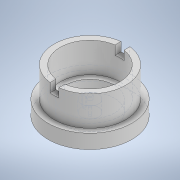
# Autodesk Inventor part: LidBottom
Saved by Autodesk Inventor 2020 (Build 240168000, 168)
## iProperties
Created: 2022-03-01
Part Number: LidBottom
Material: Generic
Document SubType Name: Modeling
Designer: atharun
Density: 1 g/cm^3
Appearance: Default
Mass: 115.288 g
Surface Area: 338.563 cm^2
Volume: 115.288 cm^3
Author: atharun
Autodesk Inventor part; units mm, degrees
sketch "Sketch1" plane through (0, 0, 0) normal (0, 1, 0) x (-1, 0, 0)
  circle A0 centre (0, 0) radius 44.45
  circle A1 centre (0, 0) radius 6.75
  dimension "d0" = 88.9
  dimension "d3" = 13.5
  constraints: 2 centre point, 2 coincident
  measures "d0" diameter of A0
  measures "d3" diameter of A1
extrude "Extrusion2" add sketch "Sketch1" along normal blind 2 contours A0 | A1
sketch "Sketch2" plane through (0, 2, 0) normal (0, 1, 0) x (1, 0, 0)
  circle A0 centre (0, 0) radius 10
  circle A1 centre (0, 0) radius 44.45
  dimension "d6" = 20
  dimension "d37" = 88.9
  constraints: 2 centre point, 2 coincident
  measures "d6" diameter of A0
  measures "d37" diameter of A1
extrude "Extrusion3" add sketch "Sketch2" along normal blind 7 contours A0 | A1
sketch "Sketch3" plane through (0, 9, 0) normal (0, 1, 0) x (1, 0, 0)
  circle A0 centre (0, 0) radius 44.45
  dimension "d9" = 88.9
  constraints: 1 centre point, 1 coincident
  measures "d9" diameter of A0
extrude "Extrusion4" add sketch "Sketch3" along normal blind 6
sketch "Sketch4" plane through (0, 15, 0) normal (0, 1, 0) x (1, 0, 0)
  circle A0 centre (0, 0) radius 38.0048
  circle A1 centre (0, 0) radius 31.75
  point P0 (-38.0048, 0)
  point P1 (0, 38.0048)
  point P2 (38.0048, 0)
  point P3 (0, -38.0048)
  dimension "d12" = 76.0095
  dimension "d13" = 63.5
  constraints: 4 point on circle, 2 centre point, 2 coincident
  measures "d12" diameter of A0
  measures "d13" diameter of A1
extrude "Extrusion5" add sketch "Sketch4" along normal blind 31.75
ref_plane "Work Plane3" through (38.0048, 15, 0) normal (1, 0, 0) x (0, 1, 0)
ref_plane "Work Plane4" through (-38.0048, 15, 0) normal (-1, 0, 0) x (0, -1, 0)
sketch "Sketch8" plane through (38.0048, 15, 0) normal (1, 0, 0) x (0, 1, 0)
  line L0 (31.75, -38.0048) -> (31.75, 38.0048) projected
  line L1 (31.75, 6.35) -> (14.224, 6.35)
  line L2 (14.224, 6.35) -> (14.224, -6.35)
  line L3 (14.224, -6.35) -> (31.75, -6.35)
  line L4 (31.75, -6.35) -> (31.75, 6.35)
  line L5 (31.75, 0) -> (0, 0)
  line L6 (0, -44.45) -> (0, 44.45) projected
  line L7 (21.844, 5.08) -> (17.4498, 5.08)
  line L8 (17.4498, 5.08) -> (17.4498, -5.08)
  line L9 (17.4498, -5.08) -> (21.844, -5.08)
  line L10 (21.844, -5.08) -> (21.844, 5.08)
  line L11 (25.146, 6.35) -> (25.146, -6.35)
  point P0 (-15, 0)
  dimension "d38" = 17.526
  dimension "d39" = 12.7
  dimension "d41" = 6.35
  dimension "d42" = 9.906
  dimension "d43" = 10.16
  dimension "d44" = 5.08
  dimension "d46" = 4.3942
  dimension "d70" = 6.604
  constraints: 20 end point, 4 parallel, 3 perpendicular, 3 point on line, 2 horizontal, 2 midpoint
  measures "d38" distance of L3.end L2.end
  measures "d39" distance of L2.end L1.end
  measures "d41" distance between parallel lines of L1 L5
  measures "d42" distance between parallel lines of L10 L0
  measures "d43" distance of L7.end L8.end
  measures "d44" distance between parallel lines of L5 L9
  measures "d46" distance of L7.start L7.end
  measures "d70" distance between parallel lines of L0 L11
extrude "Extrusion9" [suppressed]
ref_plane "Work Plane5" through (0, 15, 0) normal (-1, 0, 0) x (0, -1, 0)
mirror "Mirror1" [suppressed]
fillet "Fillet3" [suppressed]
fillet "Fillet4" [suppressed]
fillet "Fillet5" [suppressed]
fillet "Fillet6" [suppressed]
sketch "Sketch9" plane through (0, 15, 0) normal (0, 1, 0) x (1, 0, 0)
  line L0 (-9, 0.8983) -> (-5, 0.8983)
  line L1 (-9.0449, -0.0017) -> (-5, -0.0017)
  line L2 (-5, -0.0017) -> (-5, 0.8983)
  circle A0 centre (0, -0.0017) radius 9.0449
  circle A1 centre (0, -0.0017) radius 21.8449
  line L3 (-21.8449, 0) -> (-25.8449, 0)
  circle A2 centre (0, -0.0017) radius 25.8449
  point P0 (0, 0)
  dimension "d62" = 43.6898
  dimension "d57" = 4
  dimension "d58" = 5
  dimension "d60" = 0.9
  dimension "x" = 18.0898
  dimension "d63" = 4
  constraints: 8 end point, 3 coincident, 3 horizontal, 2 point on circle, 1 centre point, 1 perpendicular, 6 other
  measures "d57" distance of L0.start L0.end
  measures "d58" horizontal distance of point (0, 0) L0.end
  measures "d60" distance of L1.end L0.end
  measures "x" diameter of A0
  measures "d63" distance of L3.start L3.end
extrude "Extrusion10" cut sketch "Sketch9" against normal blind 12 contours L0 L2 L1 A0 | A1 | A2 picked at (-6.3416, 0.4985)
sketch "Sketch10" plane through (0, 15, 0) normal (0, 1, 0) x (1, 0, 0)
  circle A0 centre (0, 0) radius 2.3178
  dimension "d67" = 4.6355
  constraints: 1 centre point, 1 coincident
  measures "d67" diameter of A0
extrude "Extrusion11" add sketch "Sketch10" along normal blind 4.064
ref_plane "Work Plane6" through (0, 15, 38.0048) normal (0, 0, 1) x (1, 0, 0)
sketch "Sketch11" plane through (0, 15, 38.0048) normal (0, 0, 1) x (1, 0, 0)
  line L0 (-31.75, 31.75) -> (31.75, 31.75) projected
  line L1 (0, 31.75) -> (0, 22.225)
  line L2 (-4.7625, 22.225) -> (4.7625, 22.225)
  line L3 (4.7625, 22.225) -> (4.7625, 31.75)
  line L4 (4.7625, 31.75) -> (-4.7625, 31.75)
  line L5 (-4.7625, 31.75) -> (-4.7625, 22.225)
  point P0 (0, -15)
  point P1 (-4.7625, 31.75)
  dimension "d71" = 9.525
  dimension "d72" = 4.7625
  dimension "d73" = 4.7625
  constraints: 10 end point, 2 parallel, 1 horizontal, 1 midpoint, 1 perpendicular, 1 point on line, 1 vertical
  measures "d71" distance of L1.start L1.end
  measures "d72" distance between parallel lines of L1 L5
  measures "d73" distance between parallel lines of L3 L1
extrude "Extrusion12" cut sketch "Sketch11" against normal blind 100.0872
sketch "Sketch12" plane through (0, 0, 0) normal (0, -1, 0) x (1, 0, 0)
  circle A0 centre (0, 0) radius 1.5
  dimension "d76" = 3
  constraints: 1 centre point, 1 coincident
  measures "d76" diameter of A0
extrude "Extrusion13" cut sketch "Sketch12" against normal blind 8
thread "Thread2" size "M3x0.5" class "6H" standard "ANSI Metric M Profile" full length
body "Solid2"
